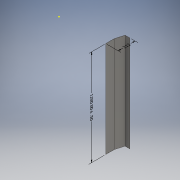
# Autodesk Inventor part: front
Saved by Autodesk Inventor 2018 (Build 220112000, 112)
## iProperties
Created: 2018-04-10
Part Number: front
Material: Steel
Document SubType Name: Modeling
Designer: P446509
Density: 7.85 g/cm^3
Appearance: Stainless - Brushed
Author: P446509
Autodesk Inventor part; units mm, degrees
ref_plane "YZ Plane" through (0, 0, 0) normal (1, 0, 0) x (0, 1, 0)
ref_plane "XZ Plane" through (0, 0, 0) normal (0, 1, 0) x (-1, 0, 0)
ref_plane "XY Plane" through (0, 0, 0) normal (0, 0, 1) x (1, 0, 0)
sketch "Sketch1" plane through (0, 0, 0) normal (0, 0, 1) x (1, 0, 0)
  line L0 (583, 0) -> (583, -566) projected
  line L1 (613.4835, 107.0681) -> (1060.6433, 107.0681) projected
  point P0 (0, 0)
  constraints: 2 coincident
sketch "Sketch2" plane through (0, 0, 0) normal (0, 0, 1) x (1, 0, 0)
  line L0 (583, 0) -> (613.4835, 107.0681)
  line L1 (613.4835, 107.0681) -> (673.4835, 107.0681)
  line L2 (583, 0) -> (583, -105)
  line L3 (673.4835, 105.4681) -> (614.6916, 105.4681)
  line L4 (614.6916, 105.4681) -> (584.6, -0.2233)
  line L5 (584.6, -0.2233) -> (584.6, -105)
  line L6 (583, -105) -> (584.6, -105)
  line L7 (673.4835, 107.0681) -> (673.4835, 105.4681)
  point P0 (0, 0)
  dimension "d0" = 105
  dimension "d1" = 60
  dimension "d2" = 1.6
  constraints: 16 end point, 2 horizontal, 1 perpendicular, 1 vertical, 2 other
  measures "d0" distance of L0.start L2.end
  measures "d1" distance of L0.end L1.end
  measures "d2" distance between parallel lines of L0 L4
extrude "Extrusion1" add sketch "Sketch2" against normal blind 1200
sketch "Sketch3" plane through (583, -105, -1200) normal (0, -1, 0) x (1, 0, 0)
  point P0 (-583, 1200)
body "Solid1"
